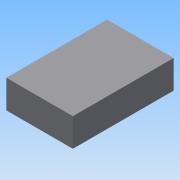
# Autodesk Inventor part: Scale
Saved by Autodesk Inventor 2016 (Build 200138000, 138)
## iProperties
Created: 2014-11-14
Part Number: Scale
Material: Blei
Document SubType Name: Modeling
Designer: Gero Hofmann
Density: 11.37 g/cm^3
Appearance: Blei
Author: Gero Hofmann
Autodesk Inventor part; units mm, degrees
ref_plane "YZ Plane" through (0, 0, 0) normal (1, 0, 0) x (0, 1, 0)
ref_plane "XZ Plane" through (0, 0, 0) normal (0, 1, 0) x (-1, 0, 0)
ref_plane "XY Plane" through (0, 0, 0) normal (0, 0, 1) x (1, 0, 0)
sketch "Skizze1" plane through (0, 0, 0) normal (0, 0, 1) x (1, 0, 0)
  line L0 (-82.5, 125) -> (82.5, 125)
  line L1 (82.5, 125) -> (82.5, -125)
  line L2 (82.5, -125) -> (-82.5, -125)
  line L3 (-82.5, -125) -> (-82.5, 125)
  line L4 (-82.5, 125) -> (82.5, -125) construction
  line L5 (82.5, 125) -> (-82.5, -125) construction
  point P0 (0, 0)
  dimension "d0" = 165
  dimension "d1" = 250
  constraints: 12 end point, 2 midpoint, 2 parallel, 1 horizontal, 1 perpendicular
  measures "d0" distance of L1.end L2.end
  measures "d1" distance of L0.end L1.end
extrude "Extrusion1" add sketch "Skizze1" along normal blind 70
sketch "Skizze2" plane through (0, 0, 0) normal (0, 0, -1) x (-1, 0, 0)
  line L0 (82.5, 125) -> (-82.5, 125) projected
  circle A0 centre (0, 37.5) radius 52.5
  point P0 (0, 0)
  dimension "d4" = 105
  dimension "d5" = 35
  constraints: 1 centre point
  measures "d4" diameter of A0
  measures "d5" distance edge to line of A0 L0
extrude "Extrusion2" add sketch "Skizze2" along normal blind 10
chamfer "Fase1" distance 30 angle 60 1 edges at (0, -125, 0) measured on face at (27.5, -125, 23.3333)
sketch "Skizze3" plane through (0, 0, 70) normal (0, 0, 1) x (1, 0, 0)
  line L0 (82.5, 125) -> (-82.5, 125) projected
  line L1 (-82.5, 125) -> (-82.5, -125) projected
  line L2 (-82.5, -125) -> (82.5, -125) projected
  line L3 (82.5, -125) -> (82.5, 125) projected
  line L4 (-82.5, -115) -> (82.5, -115)
  point P0 (0, 0)
  dimension "d11" = 10
  constraints: 2 end point, 2 point on line, 1 perpendicular
  measures "d11" distance between parallel lines of L2 L4
ref_plane "Arbeitsebene1" through (-82.5, -115, 70) normal (0, 0.1736, 0.9848) x (1, 0, 0)
sketch "Skizze4" plane through (0, 0, 70) normal (0, 0, 1) x (1, 0, 0)
  line L0 (82.5, 125) -> (-82.5, 125) projected
  line L1 (-82.5, 125) -> (-82.5, -125) projected
  line L2 (82.5, -125) -> (82.5, 125) projected
  line L3 (-70, -115) -> (70, -115) construction
  line L4 (70, -115) -> (70, 115)
  line L5 (70, 115) -> (-70, 115)
  line L6 (-70, 115) -> (-70, -115)
  line L7 (-70, -115) -> (70, 115) construction
  line L8 (70, -115) -> (-70, 115) construction
  line L9 (-82.5, -115) -> (82.5, -115) projected
  point P0 (0, 0)
  point P1 (0, 0)
  point P2 (0, 0)
  dimension "d13" = 230
  dimension "d14" = 140
  constraints: 12 end point, 3 midpoint, 2 coincident, 2 parallel, 2 point on line, 1 horizontal, 1 perpendicular
  measures "d13" distance of L3.end L4.end
  measures "d14" distance of L4.end L5.end
extrude "Extrusion3" cut sketch "Skizze4" against normal up to surface contours L2 L9 L4 L5 L6 L1 L0 surface through (-82.5, -115, 70) normal (0, 0.1736, 0.9848)
sketch "Skizze5" plane through (0, 0, 70) normal (0, 0, 1) x (1, 0, 0)
  line L0 (82.5, -115) -> (70, -115) projected
  line L1 (70, -115) -> (70, 115) projected
  line L2 (70, 115) -> (-70, 115) projected
  line L3 (-70, 115) -> (-70, -115) projected
  line L4 (-70, -115) -> (-82.5, -115) projected
  line L5 (-82.5, -115) -> (-82.5, -125) projected
  line L6 (-82.5, -125) -> (82.5, -125) projected
  line L7 (82.5, -125) -> (82.5, -115) projected
  line L8 (55, 100) -> (-55, 100) construction
  line L9 (-55, 100) -> (-55, -100) construction
  line L10 (-55, -100) -> (55, -100) construction
  line L11 (55, -100) -> (55, 100) construction
  line L12 (55, 100) -> (-55, -100) construction
  line L13 (-55, 100) -> (55, -100) construction
  circle A0 centre (-55, -100) radius 15
  circle A1 centre (-55, 100) radius 15
  circle A2 centre (55, 100) radius 15
  circle A3 centre (55, -100) radius 15
  line L14 (-82.5, -115) -> (-82.5, 125) projected
  line L15 (-70, -115) -> (-82.5, -115) projected
  line L16 (-70, 115) -> (-70, -115) projected
  line L17 (70, 115) -> (-70, 115) projected
  line L18 (70, -115) -> (70, 115) projected
  line L19 (82.5, -115) -> (70, -115) projected
  line L20 (82.5, 125) -> (82.5, -115) projected
  line L21 (-82.5, 125) -> (82.5, 125) projected
  point P0 (0, 0)
  dimension "d17" = 110
  dimension "d18" = 200
  dimension "d19" = 30
  constraints: 12 end point, 4 centre point, 4 coincident, 3 equal radius, 2 midpoint, 2 parallel, 1 horizontal, 1 perpendicular
  measures "d17" distance of L10.end L9.end
  measures "d18" distance of L9.end L8.end
  measures "d19" diameter of A0
extrude "Extrusion4" cut sketch "Skizze5" against normal blind 5 contours L7 L6 L5 L4 L3 A1 L2 A2 L1 L0 | L0 L1 L2 L3 L4 L14 L21 L20 | A2 L2 L1 | A1 L3 L2
